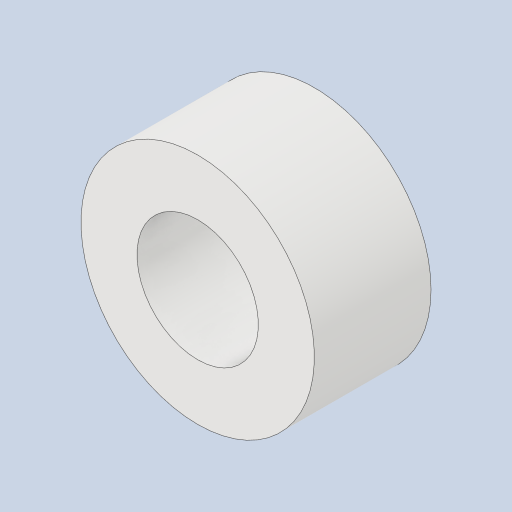
# Autodesk Inventor part: FWSJJ-D5-V2_6-T2_5
Saved by Autodesk Inventor 2023 (Build 270158000, 158)
## iProperties
Category: PARTsolutions
Company: MISUMI
Created: 2024-11-14
Part Number: FWSJJ-D5-V2_6-T2_5
Material: Generic
Catalog Web Link: www.cadenas.de
Description: FWSJJ, FWSJK, FWSJM, FWSJW, FWSJD, FWSJB, FWSJN-Resin Washers - Configurable
Vendor: MISUMI
Document SubType Name: Modeling
Designer: psAdmin
Manufacturer: MISUMI
Mass: 0.0644655 g
Surface Area: 1.36094 cm^2
Volume: 0.0644655 cm^3
Density: 1 g/cm^3
Appearance: PSOLRGB-255-255-255
PSOL_IDENT_0: {$CADENAS_DATA/23d-libs/misumi/metric/26_washers_collars/fwsjb.prj},247 {VTYP=3D},{NB=FWSJJ-D5-V2.6-
PSOL_IDENT_1: T4.5},{LINA=FWSJJ-D5-V2.6-T4.5},{NN=FWSJJ, FWSJK, FWSJM, FWSJW, FWSJD, FWSJB, FWSJN},{DATE=29.05.202
PSOL_IDENT_2: 3 07:54:15},{GEOMDATE=27.02.2019 05:03:52},{VERSION=},{LINEID=10},{WBVAR=MAT,COLOR,D,V,T,ALT1,ALT2},
PSOL_IDENT_3: {WBNUMERIC=D,V,T}  {NB=FWSJJ-D5-V2.6-T4.5},{LINA=FWSJJ-D5-V2.6-T4.5},{KT=DUMMY},{PN=FWSJJ-D5-V2.6-T4
PSOL_IDENT_4: .5},{TYPE=FWSJJ},{MAT=1},{COLOR=W},{D=5.0},{DA=[4:20/0.5],[21:100/1]},{V=2.6},{VA=0,2,2.6,[3:3/0.5]}
PSOL_IDENT_5: ,{T=4.5},{D2=3.000},{D6=-1.000},{COLOR1='W','White','B','Black'},{COLOR2=1.00,1.00,1.00,0.00},{ALT1=
PSOL_IDENT_6: },{ALT1A= '','N/A' },{ALT2=},{ALT2A= '','N/A' }
NB: FWSJJ-D5-V2.6-T4.5
NN: FWSJJ, FWSJK, FWSJM, FWSJW, FWSJD, FWSJB, FWSJN
NT: Resin Washers - Configurable
NBSYN: $PN.
LINA: FWSJJ-D5-V2.6-T4.5
CATALOG: Misumi
PN: FWSJJ-D5-V2.6-T4.5
MAT: Polyacetal
COLOR: White
D: 5
V: 2.6
T: 4.5
ALT1: N/A
ALT2: N/A
SUPPLIER: MISUMI
ARTICLENO: FWSJJ-D5-V2.6-T4.5
BOMINFO: FWSJJ-D5-V2.6-T4.5
CREATOR: CADENAS GmbH
Title: FWSJJ-D5-V2.6-T4.5
Author: Cadenas PARTsolutions
Comments: Resin Washers - Configurable
Autodesk Inventor part; units mm, degrees
ref_plane "YZ Plane" through (0, 0, 0) normal (1, 0, 0) x (0, 1, 0)
ref_plane "XZ Plane" through (0, 0, 0) normal (0, 1, 0) x (-1, 0, 0)
ref_plane "XY Plane" through (0, 0, 0) normal (0, 0, 1) x (1, 0, 0)
sketch "Sketch_1" plane through (0, 0, 0) normal (0, 0, 1) x (1, 0, 0)
  line L0 (0, 0) -> (4.5, 0)
  line L1 (4.5, 0) -> (4.5, -2.5)
  line L2 (4.5, -2.5) -> (0, -2.5)
  line L3 (0, -2.5) -> (0, 0)
  line L4 (0, 0) -> (4.5, 0)
  constraints: 10 end point
revolve "Revolution1" add sketch "Sketch_1" angle 360 about axis through (0, 0, 0) along (-1, 0, 0)
sketch "Sketch2" plane through (0, 0, 0) normal (-1, 0, 0) x (0, 0, 1)
  point P0 (0, 0)
hole "Hole1" at (0, 0, 0) direction (1, 0, 0) diameter 2.6 depth 4.5
sketch "スケッチ3" plane through (4.5, 0, 0) normal (1, 0, 0) x (0, 0, -1)
  circle A0 centre (0, 0) radius 1.3
  circle A1 centre (0, 0) radius 2.5
  constraints: 2 centre point, 2 coincident
extrude "押し出し1" cut sketch "スケッチ3" against normal blind 2
body "Solid1"
